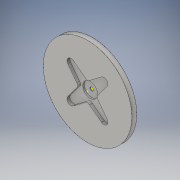
# Autodesk Inventor part: Aidan Sherry Wheel
Saved by Autodesk Inventor 2016 (Build 200138000, 138)
## iProperties
Created: 2016-10-14
Part Number: Aidan Sherry Wheel
Material: Generic
Document SubType Name: Modeling
Designer: sherra
Density: 1 g/cm^3
Appearance: Default
Author: sherra
Autodesk Inventor part; units mm, degrees
ref_plane "YZ Plane" through (0, 0, 0) normal (1, 0, 0) x (0, 1, 0)
ref_plane "XZ Plane" through (0, 0, 0) normal (0, 1, 0) x (-1, 0, 0)
ref_plane "XY Plane" through (0, 0, 0) normal (0, 0, 1) x (1, 0, 0)
sketch "Sketch1" plane through (0, 0, 0) normal (0, 0, 1) x (1, 0, 0)
  circle A0 centre (0, 0) radius 31.5468
  dimension "d0" = 63.0936
  constraints: 1 centre point, 1 coincident
  measures "d0" diameter of A0
extrude "Extrusion1" add sketch "Sketch1" along normal blind 3.556
sketch "Sketch5" plane through (0, 0, 3.556) normal (0, 0, 1) x (1, 0, 0)
  arc A0 (1.5256, -7.6067) -> (-1.5256, -7.6067) centre (0, -8.5367) ccw
  line L0 (1.5256, -7.6067) -> (10.0877, -14.0155)
  arc A1 (10.0877, -14.0155) -> (14.0155, -10.0877) centre (11.7691, -11.7691) ccw
  line L1 (14.0155, -10.0877) -> (7.6067, -1.5256)
  arc A2 (7.6067, 1.5256) -> (7.6067, -1.5256) centre (8.5367, 0) ccw
  line L2 (7.6067, 1.5256) -> (14.0155, 10.0877)
  arc A3 (14.0155, 10.0877) -> (10.0877, 14.0155) centre (11.7691, 11.7691) ccw
  line L3 (10.0877, 14.0155) -> (1.5256, 7.6067)
  arc A4 (-1.5256, 7.6067) -> (1.5256, 7.6067) centre (0, 8.5367) ccw
  line L4 (-1.5256, 7.6067) -> (-10.0877, 14.0155)
  arc A5 (-10.0877, 14.0155) -> (-14.0155, 10.0877) centre (-11.7691, 11.7691) ccw
  line L5 (-14.0155, 10.0877) -> (-7.6067, 1.5256)
  arc A6 (-7.6067, -1.5256) -> (-7.6067, 1.5256) centre (-8.5367, 0) ccw
  line L6 (-7.6067, -1.5256) -> (-14.0155, -10.0877)
  arc A7 (-14.0155, -10.0877) -> (-10.0877, -14.0155) centre (-11.7691, -11.7691) ccw
  line L7 (-10.0877, -14.0155) -> (-1.5256, -7.6067)
  circle A8 centre (12.339, -12.339) radius 0.75
  circle A9 centre (9.8641, -9.8641) radius 0.75
  circle A10 centre (7.3893, -7.3893) radius 0.75
  circle A11 centre (4.9144, -4.9144) radius 0.75
  circle A12 centre (12.339, 12.339) radius 0.75
  circle A13 centre (9.8641, 9.8641) radius 0.75
  circle A14 centre (7.3893, 7.3893) radius 0.75
  circle A15 centre (4.9144, 4.9144) radius 0.75
  circle A16 centre (-12.339, 12.339) radius 0.75
  circle A17 centre (-9.8641, 9.8641) radius 0.75
  circle A18 centre (-7.3893, 7.3893) radius 0.75
  circle A19 centre (-4.9144, 4.9144) radius 0.75
  circle A20 centre (-12.339, -12.339) radius 0.75
  circle A21 centre (-9.8641, -9.8641) radius 0.75
  circle A22 centre (-7.3893, -7.3893) radius 0.75
  circle A23 centre (-4.9144, -4.9144) radius 0.75
  circle A24 centre (0, 0) radius 3.6
  constraints: 25 centre point, 16 end point, 16 point on circle
extrude "Extrusion4" cut sketch "Sketch5" against normal blind 1.9558 contours A0 L7 A7 L6 A6 L5 A5 L4 A4 L3 A3 L2 A2 L1 A1 L0 | A8 | A9 | A10 | A11 | A12 | A13 | A14 | A15 | A16 | A17 | A18 | A19 | A20 | A21 | A22 | A23 | A24
sketch "Sketch6" plane through (0, 0, 0) normal (0, 1, 0) x (-1, 0, 0)
  point P0 (0, 0)
sketch "Sketch7" plane through (0, 0, 0) normal (0, 1, 0) x (-1, 0, 0)
  point P0 (0, 0)
sketch "Sketch8" plane through (0, 0, 0) normal (1, 0, 0) x (0, 1, 0)
  line L0 (31.5468, 0) -> (31.5468, 3.556) projected
  circle A0 centre (31.5468, 1.778) radius 1.7361
  line L1 (0, 0) -> (0, 3.556)
  line L2 (31.5468, 3.556) -> (-31.5468, 3.556) projected
  constraints: 2 end point, 2 midpoint, 1 centre point
revolve "Revolution1" cut sketch "Sketch8" angle 360 about axis through (0, 0, 0) along (0, 0, 1)
sketch "Sketch9" plane through (0, 0, 1.6002) normal (0, 0, 1) x (1, 0, 0)
  circle A0 centre (0, 0) radius 1.27
  circle A1 centre (0, 0) radius 5.2705
  constraints: 2 centre point, 2 coincident
extrude "Extrusion5" cut sketch "Sketch9" along normal mid plane 25.4 contours A0
sketch "Sketch10" plane through (0, 0, 3.556) normal (0, 0, 1) x (1, 0, 0)
  point P0 (0, 0)
sketch "Sketch11" plane through (0, 0, 1.6002) normal (0, 0, 1) x (1, 0, 0)
  circle A0 centre (0, 0) radius 5.2705
  constraints: 1 centre point, 1 coincident
extrude "Extrusion6" cut sketch "Sketch11" against normal blind 1.016
body "Solid1"
